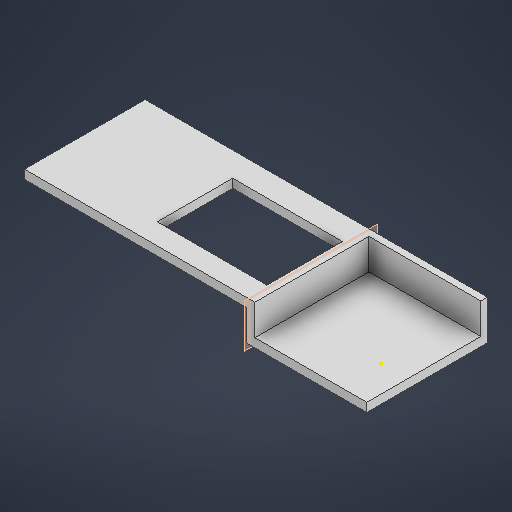
# Autodesk Inventor part: gps _mount
Saved by Autodesk Inventor 2026.1 (Build 301233000, 233)
## iProperties
Created: 2025-08-21
Part Number: gps _mount
Material: Generic
Document SubType Name: Modeling
Designer: Paweł
Density: 1 g/cm^3
Appearance: Default
Author: Paweł
Autodesk Inventor part; units mm, degrees
ref_plane "YZ Plane" through (0, 0, 0) normal (1, 0, 0) x (0, 1, 0)
ref_plane "XZ Plane" through (0, 0, 0) normal (0, 1, 0) x (-1, 0, 0)
ref_plane "XY Plane" through (0, 0, 0) normal (0, 0, 1) x (1, 0, 0)
sketch "Sketch1" plane through (0, 0, 0) normal (0, 1, 0) x (-1, 0, 0)
  line L0 (71.974, 9.2811) -> (-6.026, 9.2811)
  line L1 (-6.026, 9.2811) -> (-6.026, -18.2189)
  line L2 (-6.026, -18.2189) -> (71.974, -18.2189)
  line L3 (71.974, -18.2189) -> (71.974, 9.2811)
  point P0 (0, 0)
  dimension "d0" = 27.5
  dimension "d1" = 78
  constraints: 8 end point, 2 parallel, 1 horizontal, 1 perpendicular
  measures "d0" distance of L0.end L1.end
  measures "d1" distance of L0.start L0.end
extrude "Extrusion1" add sketch "Sketch1" along normal blind 9
sketch "Sketch2" plane through (0, 9, 0) normal (0, 1, 0) x (1, 0, 0)
  line L0 (6.026, 18.2189) -> (-71.974, 18.2189) projected
  line L1 (-71.974, -9.2811) -> (6.026, -9.2811) projected
  line L2 (6.026, 18.2189) -> (-19.474, 18.2189)
  line L3 (-19.474, 18.2189) -> (-19.474, -9.2811)
  line L4 (-19.474, -9.2811) -> (6.026, -9.2811)
  line L5 (6.026, -9.2811) -> (6.026, 18.2189)
  point P0 (0, 0)
  point P1 (6.026, -9.2811)
  point P2 (-19.474, 18.2189)
  dimension "d4" = 25.5
  constraints: 8 end point, 2 parallel, 1 horizontal, 1 perpendicular, 1 point on line
  measures "d4" distance of L4.end L3.end
extrude "Extrusion2" cut sketch "Sketch2" against normal blind 7
sketch "Sketch3" plane through (0, 2, 0) normal (0, 1, 0) x (1, 0, 0)
  point P0 (0, 0)
sketch "Sketch4" plane through (0, 2, 0) normal (0, 1, 0) x (1, 0, 0)
  line L0 (-19.474, -9.2811) -> (-19.474, 18.2189) projected
  line L1 (6.026, -9.2811) -> (6.026, 18.2189) projected
  line L2 (-19.474, 18.2189) -> (6.026, 18.2189)
  line L3 (6.026, 18.2189) -> (6.026, 16.7189)
  line L4 (6.026, 16.7189) -> (-19.474, 16.7189)
  line L5 (-19.474, 16.7189) -> (-19.474, 18.2189)
  point P0 (0, 0)
  point P1 (6.026, 18.2189)
  point P2 (-19.474, 16.7189)
  dimension "d7" = 1.5
  constraints: 8 end point, 2 parallel, 1 horizontal, 1 perpendicular, 1 point on line
  measures "d7" distance of L2.end L3.end
extrude "Extrusion3" add sketch "Sketch4" along normal blind 7
sketch "Sketch5" plane through (-71.974, 0, 9.2811) normal (0, 0, 1) x (1, 0, 0)
  line L0 (0, 9) -> (52.5, 9) projected
  line L1 (50.5, 9) -> (50.5, 0)
  line L2 (0, 0) -> (78, 0) projected
  line L3 (52.5, 2) -> (52.5, 9) projected
  line L4 (50.5, 7) -> (0, 7)
  line L5 (52.5, 2) -> (52.5, 9) projected
  line L6 (0, 9) -> (52.5, 9) projected
  line L7 (0, 0) -> (0, 9) projected
  line L8 (0, 0) -> (78, 0) projected
  line L9 (78, 0) -> (78, 2) projected
  line L10 (78, 2) -> (52.5, 2) projected
  point P0 (71.974, 0)
  point P1 (0, 7)
  dimension "d10" = 2
  dimension "d11" = 2
  constraints: 4 end point, 3 point on line, 1 horizontal, 1 vertical
  measures "d10" distance between parallel lines of L1 L3
  measures "d11" distance between parallel lines of L0 L4
extrude "Extrusion4" cut sketch "Sketch5" against normal blind 44 contours L4 L1 L2 L7
sketch "Sketch8" plane through (-71.974, 7, 9.2811) normal (0, -1, 0) x (1, 0, 0)
  line L0 (50.5, -21.9505) -> (25.5, -21.9505)
  line L1 (25.5, -21.9505) -> (25.5, -4.7505)
  line L2 (25.5, -4.7505) -> (50.5, -4.7505)
  line L3 (50.5, -4.7505) -> (50.5, -21.9505)
  line L4 (50.5, 0) -> (50.5, -27.5) projected
  point P0 (71.974, -9.2811)
  dimension "d20" = 17.2
  dimension "d21" = 25
  dimension "d22" = 0
  constraints: 8 end point, 2 parallel, 1 horizontal, 1 perpendicular
  measures "d20" distance of L0.end L1.end
  measures "d21" distance of L1.end L2.end
  measures "d22" distance between parallel lines of L4 L3
extrude "Extrusion6" cut sketch "Sketch8" against normal blind 2
ref_plane "Work Plane1" through (-20.474, 2, 9.2811) normal (1, 0, 0) x (0, 0, -1)
body "Solid1"
